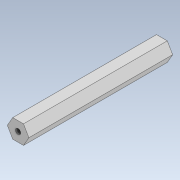
# Autodesk Inventor part: M1-Standoff-20mm
Saved by Autodesk Inventor 2020 (Build 240168000, 168)
## iProperties
Created: 2021-07-13
Part Number: M1-Standoff-20mm
Material: Generic
Document SubType Name: Modeling
Designer: Val
Density: 1 g/cm^3
Appearance: Default
Author: Val
Autodesk Inventor part; units mm, degrees
ref_plane "YZ Plane" through (0, 0, 0) normal (1, 0, 0) x (0, 1, 0)
ref_plane "XZ Plane" through (0, 0, 0) normal (0, 1, 0) x (-1, 0, 0)
ref_plane "XY Plane" through (0, 0, 0) normal (0, 0, 1) x (1, 0, 0)
sketch "Base" plane through (0, 0, 0) normal (0, 0, 1) x (1, 0, 0)
  circle A0 centre (0, 0) radius 1.5 construction
  circle A1 centre (0, 0) radius 1.5 construction
  line L0 (0.75, 1.299) -> (1.5, 0)
  line L1 (1.5, 0) -> (0.75, -1.299)
  line L2 (0.75, -1.299) -> (-0.75, -1.299)
  line L3 (-0.75, -1.299) -> (-1.5, 0)
  line L4 (-1.5, 0) -> (-0.75, 1.299)
  line L5 (-0.75, 1.299) -> (0.75, 1.299)
  line L6 (-2.1, 0) -> (2.1, 0) projected
  dimension "d1" = 3
  dimension "d0" = 3
  constraints: 12 end point, 3 coincident, 1 centre point, 1 parallel, 16 other
  measures "d0" diameter of A0
extrude "BaseFeature" add sketch "Base" along normal blind 20
sketch "MountHole" plane through (0, 0, 20) normal (0, 0, 1) x (1, 0, 0)
  point P0 (0, 0)
hole "MountHoleFeature" at (0, 0, 20) direction (0, 0, -1) diameter 0.7294 end through all thread size "M1x0.25" class "6H" standard "ISO Metric profile"
body "Solid1"
